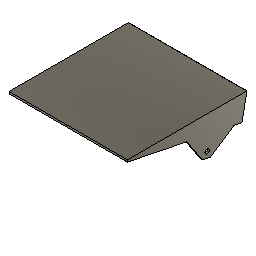
Fan Duct (Autodesk Fusion 360 design; units mm, degrees)
Autodesk Fusion 360 part; units mm, degrees
sketch "Sketch1" plane through (0, 0, 0) normal (0, 0, 1) x (1, 0, 0)
  line L0 (57, -57) -> (-57, -57)
  line L1 (-57, -57) -> (-57, 57)
  line L2 (-57, 57) -> (57, 57)
  line L3 (57, 57) -> (57, -57)
  line L4 (57, -57) -> (-57, 57) construction
  line L5 (-57, -57) -> (57, 57) construction
  dimension "d1" = 114
  dimension "d2" = 114
  constraint horizontal L0
  constraint perpendicular L0 L1
  constraint parallel L0 L2
  constraint parallel L1 L3
  constraint coincident L4 origin
  constraint coincident L5 origin
  measures "d1" distance of L1.end L2.end
  measures "d2" distance of L0.end L1.end
  measures "d21" distance of L0.start
extrude "Extrude1" add sketch "Sketch1" along normal blind 2 makes body 1
sketch "Sketch2" plane through (57, 0, 0) normal (1, 0, 0) x (0, 1, 0)
  line L0 (-57, 0) -> (57, 0)
  line L1 (57, 0) -> (57, 2)
  line L2 (57, 2) -> (-57, 2)
  line L3 (-57, 2) -> (-57, 0)
  line L4 (57, 2) -> (57, -23)
  line L5 (57, -23) -> (-57, 0)
  dimension "d5" = 25
  constraint vertical L4
  constraint coincident L1.end L2.start
  constraint coincident L0.start L3.end
  measures "d5" distance of L1.end L4.end
extrude "Extrude2" add sketch "Sketch2" along normal blind 2 separate body contours L0 L4 L5 makes body 2
extrude "Extrude3" add 1 faces at (57.6667, -19, 0) along direction (0, 0, 1) blind 2 on bodies 2 bodies 2 1
sketch "Sketch3" plane through (-57, 0, 0) normal (-1, 0, 0) x (0, -1, 0)
  line L0 (-57, 0) -> (57, 0)
  line L1 (57, 0) -> (57, 2)
  line L2 (57, 2) -> (-57, 2)
  line L3 (-57, 2) -> (-57, 0)
  line L4 (-57, 2) -> (-57, -23)
  line L5 (-57, -23) -> (57, 0)
  dimension "d10" = 25
  constraint coincident L2.end L3.start
  constraint perpendicular L2 L4
  constraint coincident L0.end L1.start
  measures "d10" distance of L2.end L4.end
extrude "Extrude4" add sketch "Sketch3" along normal blind 2 separate body contours L0 L4 L5 makes body 3
extrude "Extrude5" add 1 faces at (-57.6667, 19, 0) along direction (0, 0, 1) blind 2 on bodies 3 bodies 3 2
sketch "Sketch4" plane through (0, -2.2294, -11.0502) normal (0, -0.197769, -0.980249) x (1, 0, 0)
  line L0 (57, 55.8742) -> (57, -60.4229)
  line L1 (57, -60.4229) -> (59, -60.4229)
  line L2 (59, -60.4229) -> (59, 55.8742)
  line L3 (59, 55.8742) -> (57, 55.8742)
  line L4 (59, -60.4229) -> (57, -60.4229) construction
  line L5 (57, -60.4229) -> (57, -28.4229) construction
  line L6 (57, -28.4229) -> (59, -28.4229) construction
  line L7 (59, -28.4229) -> (59, -60.4229) construction
  line L8 (59, -24.4229) -> (57, -24.4229)
  line L9 (57, -24.4229) -> (57, -32.4229)
  line L10 (57, -32.4229) -> (59, -32.4229)
  line L11 (59, -32.4229) -> (59, -24.4229)
  line L12 (59, -24.4229) -> (57, -32.4229) construction
  line L13 (57, -24.4229) -> (59, -32.4229) construction
  point P0 (58, -28.4229)
  dimension "d15" = 32
  dimension "d16" = 2
  dimension "d17" = 8
  constraint horizontal L4
  constraint vertical L5
  constraint horizontal L6
  constraint vertical L7
  constraint coincident L0 L5.end
  constraint coincident L1.end L2.start
  constraint horizontal L8
  constraint perpendicular L8 L9
  constraint parallel L8 L10
  constraint parallel L9 L11
  constraint coincident L12 P0
  constraint coincident L13 P0
  constraint midpoint L6 P0
  measures "d15" distance of L1.end L6.end
  measures "d16" distance of L9.end L10.end
  measures "d17" distance of L8.end L9.end
extrude "Extrude6" add sketch "Sketch4" along normal blind 20 contours L0 L2 L8 L9 L10 L11 bodies 3
sketch "Sketch8" plane through (0, -2.2294, -11.0502) normal (0, -0.197769, -0.980249) x (1, 0, 0)
  line L0 (-57, -60.4229) -> (-57, 55.8742)
  line L1 (-57, 55.8742) -> (-59, 55.8742)
  line L2 (-59, 55.8742) -> (-59, -60.4229)
  line L3 (-59, -60.4229) -> (-57, -60.4229)
  line L4 (-57, -60.4229) -> (-59, -60.4229) construction
  line L5 (-59, -60.4229) -> (-59, -28.4229) construction
  line L6 (-59, -28.4229) -> (-57, -28.4229) construction
  line L7 (-57, -28.4229) -> (-57, -60.4229) construction
  line L8 (-57, -32.4229) -> (-59, -32.4229)
  line L9 (-59, -32.4229) -> (-59, -24.4229)
  line L10 (-59, -24.4229) -> (-57, -24.4229)
  line L11 (-57, -24.4229) -> (-57, -32.4229)
  line L12 (-57, -32.4229) -> (-59, -24.4229) construction
  line L13 (-59, -32.4229) -> (-57, -24.4229) construction
  point P0 (-58, -28.4229)
  dimension "d33" = 32
  dimension "d34" = 8
  constraint horizontal L4
  constraint vertical L5
  constraint horizontal L6
  constraint vertical L7
  constraint coincident L0.start L3.end
  constraint horizontal L8
  constraint perpendicular L8 L9
  constraint parallel L8 L10
  constraint parallel L9 L11
  constraint coincident L12 P0
  constraint coincident L13 P0
  constraint midpoint L6 P0
  measures "d33" distance of L0.start L6.end
  measures "d34" distance of L8.end L9.end
sketch "Sketch5" plane through (59, 0, 0) normal (1, 0, 0) x (0, 1, 0)
  line L0 (57, -23) -> (57, 2)
  line L1 (57, 2) -> (-57, 2)
  line L2 (-57, 2) -> (-57, 0)
  line L3 (-57, 0) -> (21.7111, -15.8803)
  line L4 (21.7111, -15.8803) -> (17.7557, -35.4853)
  line L5 (17.7557, -35.4853) -> (25.5977, -37.0674)
  line L6 (25.5977, -37.0674) -> (29.553, -17.4625)
  line L7 (29.553, -17.4625) -> (57, -23)
  line L8 (21.7111, -15.8803) -> (29.553, -17.4625)
  line L9 (25.632, -16.6714) -> (22.4055, -30.2945) construction
  line L10 (25.632, -16.6714) -> (39.8614, -16.6714) construction
  circle A0 centre (22.4055, -30.2945) radius 2.25
  dimension "d20" = 103.325
  dimension "d21" = 14
  dimension "d22" = 4.5
  constraint coincident L3.end L4.start
  constraint coincident L6.end L7.start
  constraint horizontal L10
  constraint midpoint L8 L9.start
  constraint coincident L9.end A0.centre
  measures "d20" angle of L9 L10
  measures "d21" distance of L9.start L9.end
  measures "d22" diameter of A0
extrude "Extrude12" add sketch "Sketch8" along normal blind 45 contours L0 L2 L8 L9 L10 L11 bodies 3
sketch "Sketch9" plane through (-59, 0, 0) normal (-1, 0, 0) x (0, -1, 0)
  line L0 (-57, 2) -> (-57, -23)
  line L1 (-57, -23) -> (-29.553, -17.4625)
  line L2 (-29.553, -17.4625) -> (-20.6534, -61.5736)
  line L3 (-20.6534, -61.5736) -> (-12.8114, -59.9915)
  line L4 (-12.8114, -59.9915) -> (-21.7111, -15.8803)
  line L5 (-21.7111, -15.8803) -> (57, 0)
  line L6 (57, 0) -> (57, 2)
  line L7 (57, 2) -> (-57, 2)
  line L8 (-29.553, -17.4625) -> (-21.7111, -15.8803) construction
  line L9 (-25.632, -16.6714) -> (-16.7324, -60.7826) construction
  circle A0 centre (-17.919, -54.9011) radius 2
  dimension "d37" = 4
  dimension "d38" = 39
  constraint coincident L1.end L2.start
  constraint coincident L4.end L5.start
  constraint midpoint L8 L9.start
  constraint midpoint L3 L9.end
  constraint coincident L9 A0.centre
  measures "d37" diameter of A0
  measures "d38" distance of L8 A0.centre
extrude "Extrude13" cut sketch "Sketch9" against normal blind 4 contours A0 bodies 3
extrude "Extrude7" cut sketch "Sketch5" against normal blind 5 contours A0 bodies 3
sketch "Sketch6" plane through (59, 0, 0) normal (1, 0, 0) x (0, 1, 0)
  circle A0 centre (22.4055, -30.2945) radius 2.25
  line L0 (57, -23) -> (57, 2)
  line L1 (57, 2) -> (-57, 2)
  line L2 (-57, 2) -> (-57, 0)
  line L3 (-57, 0) -> (21.7111, -15.8803)
  line L4 (21.7111, -15.8803) -> (17.7557, -35.4853)
  line L5 (17.7557, -35.4853) -> (25.5977, -37.0674)
  line L6 (25.5977, -37.0674) -> (29.553, -17.4625)
  line L7 (29.553, -17.4625) -> (57, -23)
  line L8 (57, -23) -> (62.2674, 3.1079)
  line L9 (57, 2) -> (62.0439, 2)
  constraint coincident L0.start L7.end
  constraint perpendicular L7 L8
  constraint coincident L0.end L1.start
  constraint coincident L8 L9.end
  constraint perpendicular L0 L9
extrude "Extrude8" add sketch "Sketch6" against normal blind 2 contours L0 L8 L9 bodies 3
sketch "Sketch7" plane through (-59, 0, 0) normal (-1, 0, 0) x (0, -1, 0)
  line L0 (-57, 2) -> (-57, -23)
  line L1 (-57, -23) -> (-29.553, -17.4625)
  line L2 (57, 0) -> (57, 2)
  line L3 (57, 2) -> (-57, 2)
  line L4 (-57, -23) -> (-62.6034, 4.7734)
  line L5 (-57, 2) -> (-62.0439, 2)
  circle A0 centre (-17.919, -54.9011) radius 2
  line L6 (-29.553, -17.4625) -> (-20.6534, -61.5736)
  line L7 (-20.6534, -61.5736) -> (-12.8114, -59.9915)
  line L8 (-12.8114, -59.9915) -> (-21.7111, -15.8803)
  line L9 (-21.7111, -15.8803) -> (57, 0)
  constraint coincident L0.end L1.start
  constraint perpendicular L1 L4
  constraint coincident L0.start L3.end
  constraint coincident L4 L5.end
  constraint perpendicular L0 L5
extrude "Extrude9" add sketch "Sketch7" against normal blind 2 contours L0 L4 L5 bodies 3
extrude "Extrude10" add 1 faces at (-19, 57, 0.6667) along direction (0, 1, 0) blind 5 on bodies 3 bodies 3
extrude "Extrude11" cut 1 faces at (-57, 61.8801, 0.5942) along direction (1, 0, 0) blind 116 on bodies 3 bodies 3
chamfer "Chamfer1" distance 20 angle 45 2 edges at (58, 29.553, -17.4625) (58, 21.7111, -15.8803) on bodies 3
chamfer "Chamfer2" distance 45 distance2 45 1 edges at (-58, 21.7111, -15.8803) measured on face at (-58.3333, -30.763, -5.2934) on bodies 3
chamfer "Chamfer3" distance 20 distance2 45 1 edges at (-58, 29.553, -17.4625) measured on face at (-57.6667, 47.851, -21.1542) on bodies 3
